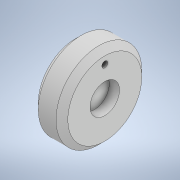
# Autodesk Inventor part: 711122
Saved by Autodesk Inventor 2022 (Build 260153000, 153)
## iProperties
Created: 2021-10-21
Part Number: 711122
Material: Типовые
Document SubType Name: Modeling
Designer: RaNSiD
Density: 1 g/cm^3
Appearance: По умолчанию
Author: RaNSiD
Autodesk Inventor part; units mm, degrees
ref_plane "YZ Plane" through (0, 0, 0) normal (1, 0, 0) x (0, 1, 0)
ref_plane "XZ Plane" through (0, 0, 0) normal (0, 1, 0) x (-1, 0, 0)
ref_plane "XY Plane" through (0, 0, 0) normal (0, 0, 1) x (1, 0, 0)
sketch "Эскиз4" plane through (0, 0, 0) normal (0, 0, 1) x (1, 0, 0)
  line L0 (0, 0) -> (-20, 0)
  line L1 (-20, 0) -> (-20, 25)
  line L2 (-16, 29) -> (-4, 29)
  line L3 (0, 25) -> (0, 0)
  line L4 (-4, 29) -> (0, 25)
  line L5 (-16, 29) -> (-20, 25)
  point P0 (-20, 29)
  point P1 (0, 29)
  dimension "d14" = 20
  dimension "d15" = 29
  dimension "d16" = 4
  dimension "d17" = 4
  dimension "d18" = 4
  dimension "d19" = 4
  constraints: 12 end point, 4 point on line, 2 parallel, 1 horizontal, 1 perpendicular
  measures "d14" distance of point (-20, 29) point (0, 29)
  measures "d15" distance of L0.end point (-20, 29)
  measures "d16" distance of L2.end point (0, 29)
  measures "d17" distance of L3.start point (0, 29)
  measures "d18" distance of L2.start point (-20, 29)
  measures "d19" distance of L1.end point (-20, 29)
revolve "Вращение3" add sketch "Эскиз4" angle 360 about axis through (0, 0, 0) along (-1, 0, 0)
sketch "Эскиз5" plane through (0, 0, 0) normal (1, 0, 0) x (0, 0, -1)
  line L0 (0, 0) -> (0, 20) construction
  dimension "d21" = 20
  constraints: 2 end point, 1 coincident, 1 vertical
  measures "d21" distance of L0.start L0.end
hole "Отверстие1" at (0, 20, 0) direction (-1, 0, 0) diameter 4 end through all
sketch "Эскиз6" plane through (0, 0, 0) normal (1, 0, 0) x (0, 0, -1)
  point P0 (0, 0)
  point P1 (0, 0)
  constraints: 1 coincident
hole "Отверстие2" at (0, 0, 0) direction (-1, 0, 0) diameter 20 depth 7
equation "\"d17\" = d16"
equation "\"d18\" = d16"
equation "\"d19\" = d18"
